Autodesk Inventor part; units mm, degrees
(part 2 of 2)
  line L911 (56.925, 86.925) -> (56.925, 75.1)
  line L912 (56.925, 75.1) -> (60.1, 75.1)
  line L913 (60.1, 75.1) -> (60.1, 64.9)
  line L914 (60.1, 64.9) -> (56.925, 64.9)
  line L915 (56.925, 64.9) -> (56.925, 55.1)
  line L916 (56.925, 55.1) -> (60.1, 55.1)
  line L917 (60.1, 55.1) -> (60.1, 44.9)
  line L918 (60.1, 44.9) -> (56.925, 44.9)
  line L919 (56.925, 44.9) -> (56.925, 35.1)
  line L920 (56.925, 35.1) -> (60.1, 35.1)
  line L921 (60.1, 35.1) -> (60.1, 24.9)
  line L922 (60.1, 24.9) -> (56.925, 24.9)
  line L923 (56.925, 24.9) -> (56.925, 15.1)
  line L924 (56.925, 15.1) -> (60.1, 15.1)
  line L925 (60.1, 15.1) -> (60.1, 4.9)
  line L926 (60.1, 4.9) -> (56.925, 4.9)
  line L927 (56.925, 4.9) -> (56.925, -4.9)
  line L928 (56.925, -4.9) -> (60.1, -4.9)
  line L929 (60.1, -4.9) -> (60.1, -15.1)
  line L930 (60.1, -15.1) -> (56.925, -15.1)
  line L931 (56.925, -15.1) -> (56.925, -24.9)
  line L932 (56.925, -24.9) -> (60.1, -24.9)
  line L933 (60.1, -24.9) -> (60.1, -35.1)
  line L934 (60.1, -35.1) -> (56.925, -35.1)
  line L935 (56.925, -35.1) -> (56.925, -44.9)
  line L936 (56.925, -44.9) -> (60.1, -44.9)
  line L937 (60.1, -44.9) -> (60.1, -55.1)
  line L938 (60.1, -55.1) -> (56.925, -55.1)
  line L939 (56.925, -55.1) -> (56.925, -64.9)
  line L940 (56.925, -64.9) -> (60.1, -64.9)
  line L941 (60.1, -64.9) -> (60.1, -75.1)
  line L942 (60.1, -75.1) -> (56.925, -75.1)
  line L943 (56.925, -75.1) -> (56.925, -86.925)
  line L944 (56.925, -86.925) -> (55.1, -86.925)
  line L945 (55.1, -86.925) -> (55.1, -90.1)
  line L946 (55.1, -90.1) -> (44.9, -90.1)
  line L947 (44.9, -90.1) -> (44.9, -86.925)
  line L948 (44.9, -86.925) -> (35.1, -86.925)
  line L949 (35.1, -86.925) -> (35.1, -90.1)
  line L950 (35.1, -90.1) -> (24.9, -90.1)
  line L951 (24.9, -90.1) -> (24.9, -86.925)
  line L952 (24.9, -86.925) -> (15.1, -86.925)
  line L953 (15.1, -86.925) -> (15.1, -90.1)
  line L954 (15.1, -90.1) -> (4.9, -90.1)
  line L955 (4.9, -90.1) -> (4.9, -86.925)
  line L956 (4.9, -86.925) -> (-4.9, -86.925)
  line L957 (-4.9, -86.925) -> (-4.9, -90.1)
  line L958 (-4.9, -90.1) -> (-15.1, -90.1)
  line L959 (-15.1, -90.1) -> (-15.1, -86.925)
  line L960 (-15.1, -86.925) -> (-24.9, -86.925)
  line L961 (-24.9, -86.925) -> (-24.9, -90.1)
  line L962 (-24.9, -90.1) -> (-35.1, -90.1)
  line L963 (-35.1, -90.1) -> (-35.1, -86.925)
  line L964 (-35.1, -86.925) -> (-44.9, -86.925)
  line L965 (-44.9, -86.925) -> (-44.9, -90.1)
  line L966 (-44.9, -90.1) -> (-55.1, -90.1)
  line L967 (-55.1, -90.1) -> (-55.1, -86.925)
  line L968 (-55.1, -86.925) -> (-56.925, -86.925)
  line L969 (-56.925, -86.925) -> (-56.925, -75.1)
  line L970 (-56.925, -75.1) -> (-60.1, -75.1)
  line L971 (-60.1, -75.1) -> (-60.1, -64.9)
  line L972 (-60.1, -64.9) -> (-56.925, -64.9)
  line L973 (-56.925, -64.9) -> (-56.925, -55.1)
  line L974 (-56.925, -55.1) -> (-60.1, -55.1)
  line L975 (-60.1, -55.1) -> (-60.1, -44.9)
  line L976 (-60.1, -44.9) -> (-56.925, -44.9)
  line L977 (-56.925, -44.9) -> (-56.925, -35.1)
  line L978 (-56.925, -35.1) -> (-60.1, -35.1)
  line L979 (-60.1, -35.1) -> (-60.1, -24.9)
  line L980 (-60.1, -24.9) -> (-56.925, -24.9)
  line L981 (-56.925, -24.9) -> (-56.925, -15.1)
  line L982 (-56.925, -15.1) -> (-60.1, -15.1)
  line L983 (-60.1, -15.1) -> (-60.1, -4.9)
  line L984 (-60.1, -4.9) -> (-56.925, -4.9)
  line L985 (-56.925, -4.9) -> (-56.925, 4.9)
  line L986 (-56.925, 4.9) -> (-60.1, 4.9)
  line L987 (-60.1, 4.9) -> (-60.1, 15.1)
  line L988 (-60.1, 15.1) -> (-56.925, 15.1)
  line L989 (-56.925, 15.1) -> (-56.925, 24.9)
  line L990 (-56.925, 24.9) -> (-60.1, 24.9)
  line L991 (-60.1, 24.9) -> (-60.1, 35.1)
  line L992 (-60.1, 35.1) -> (-56.925, 35.1)
  line L993 (-56.925, 35.1) -> (-56.925, 44.9)
  line L994 (-56.925, 44.9) -> (-60.1, 44.9)
  line L995 (-60.1, 44.9) -> (-60.1, 55.1)
  line L996 (-60.1, 55.1) -> (-56.925, 55.1)
  line L997 (-56.925, 55.1) -> (-56.925, 64.9)
  line L998 (-56.925, 64.9) -> (-60.1, 64.9)
  line L999 (-60.1, 64.9) -> (-60.1, 75.1)
  line L1000 (-60.1, 75.1) -> (-56.925, 75.1)
  line L1001 (-56.925, 75.1) -> (-56.925, 86.925)
  line L1002 (-56.925, 86.925) -> (-55.1, 86.925)
  line L1003 (-55.1, 86.925) -> (-55.1, 90.1)
  line L1004 (-55.1, 90.1) -> (-44.9, 90.1)
  line L1005 (-44.9, 90.1) -> (-44.9, 86.925)
  line L1006 (-44.9, 86.925) -> (-35.1, 86.925)
  line L1007 (-35.1, 86.925) -> (-35.1, 90.1)
  line L1008 (-35.1, 90.1) -> (-24.9, 90.1)
  line L1009 (-24.9, 90.1) -> (-24.9, 86.925)
  line L1010 (-24.9, 86.925) -> (-15.1, 86.925)
  line L1011 (-15.1, 86.925) -> (-15.1, 90.1)
  line L1012 (-14.9, 90.1) -> (-25.1, 90.1)
  line L1013 (-25.1, 90.1) -> (-25.1, 93.275)
  line L1014 (-25.1, 93.275) -> (-34.9, 93.275)
  line L1015 (-34.9, 93.275) -> (-34.9, 90.1)
  line L1016 (-34.9, 90.1) -> (-45.1, 90.1)
  line L1017 (-45.1, 90.1) -> (-45.1, 93.275)
  line L1018 (-45.1, 93.275) -> (-54.9, 93.275)
  line L1019 (-54.9, 93.275) -> (-54.9, 90.1)
  line L1020 (-54.9, 90.1) -> (-60.1, 90.1)
  line L1021 (-60.1, 90.1) -> (-60.1, 95.3)
  line L1022 (-60.1, 95.3) -> (-56.925, 95.3)
  line L1023 (-56.925, 95.3) -> (-56.925, 105.1)
  line L1024 (-56.925, 105.1) -> (-60.1, 105.1)
  line L1025 (-60.1, 105.1) -> (-60.1, 115.3)
  line L1026 (-60.1, 115.3) -> (-56.925, 115.3)
  line L1027 (-56.925, 115.3) -> (-56.925, 125.1)
  line L1028 (-56.925, 125.1) -> (-60.1, 125.1)
  line L1029 (-60.1, 125.1) -> (-60.1, 135.3)
  line L1030 (-60.1, 135.3) -> (-56.925, 135.3)
  line L1031 (-56.925, 135.3) -> (-56.925, 145.1)
  line L1032 (-56.925, 145.1) -> (-60.1, 145.1)
  line L1033 (-60.1, 145.1) -> (-60.1, 155.3)
  line L1034 (-60.1, 155.3) -> (-56.925, 155.3)
  line L1035 (-56.925, 155.3) -> (-56.925, 165.1)
  line L1036 (-56.925, 165.1) -> (-60.1, 165.1)
  line L1037 (-60.1, 165.1) -> (-60.1, 175.3)
  line L1038 (-60.1, 175.3) -> (-56.925, 175.3)
  line L1039 (-56.925, 175.3) -> (-56.925, 185.1)
  line L1040 (-56.925, 185.1) -> (-60.1, 185.1)
  line L1041 (-60.1, 185.1) -> (-60.1, 195.3)
  line L1042 (-60.1, 195.3) -> (-56.925, 195.3)
  line L1043 (-56.925, 195.3) -> (-56.925, 205.1)
  line L1044 (-56.925, 205.1) -> (-60.1, 205.1)
  line L1045 (-60.1, 205.1) -> (-60.1, 210.3)
  line L1046 (-60.1, 210.3) -> (-54.9, 210.3)
  line L1047 (-54.9, 210.3) -> (-54.9, 207.125)
  line L1048 (-54.9, 207.125) -> (-45.1, 207.125)
  line L1049 (-45.1, 207.125) -> (-45.1, 210.3)
  line L1050 (-45.1, 210.3) -> (-34.9, 210.3)
  line L1051 (-34.9, 210.3) -> (-34.9, 207.125)
  line L1052 (-34.9, 207.125) -> (-25.1, 207.125)
  line L1053 (-25.1, 207.125) -> (-25.1, 210.3)
  line L1054 (-25.1, 210.3) -> (-14.9, 210.3)
  line L1055 (-14.9, 210.3) -> (-14.9, 207.125)
  line L1056 (-14.9, 207.125) -> (-5.1, 207.125)
  line L1057 (-5.1, 207.125) -> (-5.1, 210.3)
  line L1058 (-5.1, 210.3) -> (5.1, 210.3)
  line L1059 (5.1, 210.3) -> (5.1, 207.125)
  line L1060 (5.1, 207.125) -> (14.9, 207.125)
  line L1061 (14.9, 207.125) -> (14.9, 210.3)
  line L1062 (14.9, 210.3) -> (25.1, 210.3)
  line L1063 (25.1, 210.3) -> (25.1, 207.125)
  line L1064 (25.1, 207.125) -> (34.9, 207.125)
  line L1065 (34.9, 207.125) -> (34.9, 210.3)
  line L1066 (34.9, 210.3) -> (45.1, 210.3)
  line L1067 (45.1, 210.3) -> (45.1, 207.125)
  line L1068 (45.1, 207.125) -> (54.9, 207.125)
  line L1069 (54.9, 207.125) -> (54.9, 210.3)
  line L1070 (54.9, 210.3) -> (60.1, 210.3)
  line L1071 (60.1, 210.3) -> (60.1, 205.1)
  line L1072 (60.1, 205.1) -> (56.925, 205.1)
  line L1073 (56.925, 205.1) -> (56.925, 195.3)
  line L1074 (56.925, 195.3) -> (60.1, 195.3)
  line L1075 (60.1, 195.3) -> (60.1, 185.1)
  line L1076 (60.1, 185.1) -> (56.925, 185.1)
  line L1077 (56.925, 185.1) -> (56.925, 175.3)
  line L1078 (56.925, 175.3) -> (60.1, 175.3)
  line L1079 (60.1, 175.3) -> (60.1, 165.1)
  line L1080 (60.1, 165.1) -> (56.925, 165.1)
  line L1081 (56.925, 165.1) -> (56.925, 155.3)
  line L1082 (56.925, 155.3) -> (60.1, 155.3)
  line L1083 (60.1, 155.3) -> (60.1, 145.1)
  line L1084 (60.1, 145.1) -> (56.925, 145.1)
  line L1085 (56.925, 145.1) -> (56.925, 135.3)
  line L1086 (56.925, 135.3) -> (60.1, 135.3)
  line L1087 (60.1, 135.3) -> (60.1, 125.1)
  line L1088 (60.1, 125.1) -> (56.925, 125.1)
  line L1089 (56.925, 125.1) -> (56.925, 115.3)
  line L1090 (56.925, 115.3) -> (60.1, 115.3)
  line L1091 (60.1, 115.3) -> (60.1, 105.1)
  line L1092 (60.1, 105.1) -> (56.925, 105.1)
  line L1093 (56.925, 105.1) -> (56.925, 95.3)
  line L1094 (56.925, 95.3) -> (60.1, 95.3)
  line L1095 (60.1, 95.3) -> (60.1, 90.1)
  line L1096 (60.1, 90.1) -> (54.9, 90.1)
  line L1097 (54.9, 90.1) -> (54.9, 93.275)
  line L1098 (54.9, 93.275) -> (45.1, 93.275)
  line L1099 (45.1, 93.275) -> (45.1, 90.1)
  line L1100 (45.1, 90.1) -> (34.9, 90.1)
  line L1101 (34.9, 90.1) -> (34.9, 93.275)
  line L1102 (34.9, 93.275) -> (25.1, 93.275)
  line L1103 (25.1, 93.275) -> (25.1, 90.1)
  line L1104 (25.1, 90.1) -> (14.9, 90.1)
  line L1105 (14.9, 90.1) -> (14.9, 93.275)
  line L1106 (14.9, 93.275) -> (5.1, 93.275)
  line L1107 (5.1, 93.275) -> (5.1, 90.1)
  line L1108 (5.1, 90.1) -> (-5.1, 90.1)
  line L1109 (-5.1, 90.1) -> (-5.1, 93.275)
  line L1110 (-5.1, 93.275) -> (-14.9, 93.275)
  line L1111 (-14.9, 93.275) -> (-14.9, 90.1)
  line L1112 (75.3, 90.1) -> (75.3, 86.925)
  line L1113 (75.3, 86.925) -> (85.1, 86.925)
  line L1114 (85.1, 86.925) -> (85.1, 90.1)
  line L1115 (85.1, 90.1) -> (95.3, 90.1)
  line L1116 (95.3, 90.1) -> (95.3, 86.925)
  line L1117 (95.3, 86.925) -> (105.1, 86.925)
  line L1118 (105.1, 86.925) -> (105.1, 90.1)
  line L1119 (105.1, 90.1) -> (115.3, 90.1)
  line L1120 (115.3, 90.1) -> (115.3, 86.925)
  line L1121 (115.3, 86.925) -> (125.1, 86.925)
  line L1122 (125.1, 86.925) -> (125.1, 90.1)
  line L1123 (125.1, 90.1) -> (135.3, 90.1)
  line L1124 (135.3, 90.1) -> (135.3, 86.925)
  line L1125 (135.3, 86.925) -> (145.1, 86.925)
  line L1126 (145.1, 86.925) -> (145.1, 90.1)
  line L1127 (145.1, 90.1) -> (155.3, 90.1)
  line L1128 (155.3, 90.1) -> (155.3, 86.925)
  line L1129 (155.3, 86.925) -> (165.1, 86.925)
  line L1130 (165.1, 86.925) -> (165.1, 90.1)
  line L1131 (165.1, 90.1) -> (175.3, 90.1)
  line L1132 (175.3, 90.1) -> (175.3, 86.925)
  line L1133 (175.3, 86.925) -> (180.3, 86.925)
  line L1134 (180.3, 86.925) -> (180.3, 74.9)
  line L1135 (180.3, 74.9) -> (177.125, 74.9)
  line L1136 (177.125, 74.9) -> (177.125, 65.1)
  line L1137 (177.125, 65.1) -> (180.3, 65.1)
  line L1138 (180.3, 65.1) -> (180.3, 54.9)
  line L1139 (180.3, 54.9) -> (177.125, 54.9)
  line L1140 (177.125, 54.9) -> (177.125, 45.1)
  line L1141 (177.125, 45.1) -> (180.3, 45.1)
  line L1142 (180.3, 45.1) -> (180.3, 34.9)
  line L1143 (180.3, 34.9) -> (177.125, 34.9)
  line L1144 (177.125, 34.9) -> (177.125, 25.1)
  line L1145 (177.125, 25.1) -> (180.3, 25.1)
  line L1146 (180.3, 25.1) -> (180.3, 14.9)
  line L1147 (180.3, 14.9) -> (177.125, 14.9)
  line L1148 (177.125, 14.9) -> (177.125, 5.1)
  line L1149 (177.125, 5.1) -> (180.3, 5.1)
  line L1150 (180.3, 5.1) -> (180.3, -5.1)
  line L1151 (180.3, -5.1) -> (177.125, -5.1)
  line L1152 (177.125, -5.1) -> (177.125, -14.9)
  line L1153 (177.125, -14.9) -> (180.3, -14.9)
  line L1154 (180.3, -14.9) -> (180.3, -25.1)
  line L1155 (180.3, -25.1) -> (177.125, -25.1)
  line L1156 (177.125, -25.1) -> (177.125, -34.9)
  line L1157 (177.125, -34.9) -> (180.3, -34.9)
  line L1158 (180.3, -34.9) -> (180.3, -45.1)
  line L1159 (180.3, -45.1) -> (177.125, -45.1)
  line L1160 (177.125, -45.1) -> (177.125, -54.9)
  line L1161 (177.125, -54.9) -> (180.3, -54.9)
  line L1162 (180.3, -54.9) -> (180.3, -65.1)
  line L1163 (180.3, -65.1) -> (177.125, -65.1)
  line L1164 (177.125, -65.1) -> (177.125, -74.9)
  line L1165 (177.125, -74.9) -> (180.3, -74.9)
  line L1166 (180.3, -74.9) -> (180.3, -86.925)
  line L1167 (180.3, -86.925) -> (175.3, -86.925)
  line L1168 (175.3, -86.925) -> (175.3, -90.1)
  line L1169 (175.3, -90.1) -> (165.1, -90.1)
  line L1170 (165.1, -90.1) -> (165.1, -86.925)
  line L1171 (165.1, -86.925) -> (155.3, -86.925)
  line L1172 (155.3, -86.925) -> (155.3, -90.1)
  line L1173 (155.3, -90.1) -> (145.1, -90.1)
  line L1174 (145.1, -90.1) -> (145.1, -86.925)
  line L1175 (145.1, -86.925) -> (135.3, -86.925)
  line L1176 (135.3, -86.925) -> (135.3, -90.1)
  line L1177 (135.3, -90.1) -> (125.1, -90.1)
  line L1178 (125.1, -90.1) -> (125.1, -86.925)
  line L1179 (125.1, -86.925) -> (115.3, -86.925)
  line L1180 (115.3, -86.925) -> (115.3, -90.1)
  line L1181 (115.3, -90.1) -> (105.1, -90.1)
  line L1182 (105.1, -90.1) -> (105.1, -86.925)
  line L1183 (105.1, -86.925) -> (95.3, -86.925)
  line L1184 (95.3, -86.925) -> (95.3, -90.1)
  line L1185 (95.3, -90.1) -> (85.1, -90.1)
  line L1186 (85.1, -90.1) -> (85.1, -86.925)
  line L1187 (85.1, -86.925) -> (75.3, -86.925)
  line L1188 (75.3, -86.925) -> (75.3, -90.1)
  line L1189 (75.3, -90.1) -> (65.1, -90.1)
  line L1190 (65.1, -90.1) -> (65.1, -86.925)
  line L1191 (65.1, -86.925) -> (60.1, -86.925)
  line L1192 (60.1, -86.925) -> (60.1, -74.9)
  line L1193 (60.1, -74.9) -> (63.275, -74.9)
  line L1194 (63.275, -74.9) -> (63.275, -65.1)
  line L1195 (63.275, -65.1) -> (60.1, -65.1)
  line L1196 (60.1, -65.1) -> (60.1, -54.9)
  line L1197 (60.1, -54.9) -> (63.275, -54.9)
  line L1198 (63.275, -54.9) -> (63.275, -51.4)
  line L1199 (63.275, -51.4) -> (65.475, -51.4)
  line L1200 (65.475, -51.4) -> (65.475, -52.65)
  line L1201 (65.475, -52.65) -> (67.775, -52.65)
  line L1202 (67.775, -52.65) -> (67.775, -51.4)
  line L1203 (67.775, -51.4) -> (74.1, -51.4)
  line L1204 (74.1, -51.4) -> (74.1, -48.6)
  line L1205 (74.1, -48.6) -> (67.775, -48.6)
  line L1206 (67.775, -48.6) -> (67.775, -47.35)
  line L1207 (67.775, -47.35) -> (65.475, -47.35)
  line L1208 (65.475, -47.35) -> (65.475, -48.6)
  line L1209 (65.475, -48.6) -> (63.275, -48.6)
  line L1210 (63.275, -48.6) -> (63.275, -45.1)
  line L1211 (63.275, -45.1) -> (60.1, -45.1)
  line L1212 (60.1, -45.1) -> (60.1, -34.9)
  line L1213 (60.1, -34.9) -> (63.275, -34.9)
  line L1214 (63.275, -34.9) -> (63.275, -25.1)
  line L1215 (63.275, -25.1) -> (60.1, -25.1)
  line L1216 (60.1, -25.1) -> (60.1, -14.9)
  line L1217 (60.1, -14.9) -> (63.275, -14.9)
  line L1218 (63.275, -14.9) -> (63.275, -5.1)
  line L1219 (63.275, -5.1) -> (60.1, -5.1)
  line L1220 (60.1, -5.1) -> (60.1, 5.1)
  line L1221 (60.1, 5.1) -> (63.275, 5.1)
  line L1222 (63.275, 5.1) -> (63.275, 14.9)
  line L1223 (63.275, 14.9) -> (60.1, 14.9)
  line L1224 (60.1, 14.9) -> (60.1, 25.1)
  line L1225 (60.1, 25.1) -> (63.275, 25.1)
  line L1226 (63.275, 25.1) -> (63.275, 34.9)
  line L1227 (63.275, 34.9) -> (60.1, 34.9)
  line L1228 (60.1, 34.9) -> (60.1, 45.1)
  line L1229 (60.1, 45.1) -> (63.275, 45.1)
  line L1230 (63.275, 45.1) -> (63.275, 48.6)
  line L1231 (63.275, 48.6) -> (65.475, 48.6)
  line L1232 (65.475, 48.6) -> (65.475, 47.35)
  line L1233 (65.475, 47.35) -> (67.775, 47.35)
  line L1234 (67.775, 47.35) -> (67.775, 48.6)
  line L1235 (67.775, 48.6) -> (74.1, 48.6)
  line L1236 (74.1, 48.6) -> (74.1, 51.4)
  line L1237 (74.1, 51.4) -> (67.775, 51.4)
  line L1238 (67.775, 51.4) -> (67.775, 52.65)
  line L1239 (67.775, 52.65) -> (65.475, 52.65)
  line L1240 (65.475, 52.65) -> (65.475, 51.4)
  line L1241 (65.475, 51.4) -> (63.275, 51.4)
  line L1242 (63.275, 51.4) -> (63.275, 54.9)
  line L1243 (63.275, 54.9) -> (60.1, 54.9)
  line L1244 (60.1, 54.9) -> (60.1, 65.1)
  line L1245 (60.1, 65.1) -> (63.275, 65.1)
  line L1246 (63.275, 65.1) -> (63.275, 74.9)
  line L1247 (63.275, 74.9) -> (60.1, 74.9)
  line L1248 (60.1, 74.9) -> (60.1, 86.925)
  line L1249 (60.1, 86.925) -> (65.1, 86.925)
  line L1250 (65.1, 86.925) -> (65.1, 90.1)
  line L1251 (65.1, 90.1) -> (75.3, 90.1)
  line L1252 (43.7, -59.9) -> (43.7, 59.9)
  line L1253 (43.7, 59.9) -> (-43.7, 59.9)
  line L1254 (-43.7, 59.9) -> (-43.7, -59.9)
  line L1255 (-43.7, -59.9) -> (43.7, -59.9)
  circle A22 centre (-67.924, -59.1479) radius 1.078 projected
  circle A23 centre (-102.924, -59.1479) radius 1.078 projected
  point P0 (0, 0)
  dimension "d8" = 0.1
  dimension "d9" = 0.1
  dimension "d10" = 0.1
  dimension "d11" = 0.1
  dimension "d12" = 0.1
  dimension "d13" = 0.1
  dimension "d14" = 0.1
  dimension "d15" = 0.1
  constraints: 1248 end point, 616 other
  measures "d8" distance between parallel lines of L8 L632
  measures "d9" distance between parallel lines of L0 L748
  measures "d10" distance between parallel lines of L6 L752
  measures "d11" distance between parallel lines of L188 L756
  measures "d12" distance between parallel lines of L377 L896
  measures "d13" distance between parallel lines of L448 L1012
  measures "d14" distance between parallel lines of L589 L1112
  measures "d15" distance between parallel lines of L268 L1252
extrude "Extrusion2" add sketch "Sketch2" along normal blind 3.175 contours L632 L633 L634 L635 L636 L637 L638 L639 L640 L641 L642 L643 L644 L645 L646 L647 L648 L649 L650 L651 L652 L653 L654 L655 L656 L657 L658 L659 L660 L661 L662 L663 L664 L665 L666 L667 L668 L669 L670 L671 L672 L673 L674 L675 L676 L677 L678 L679 L680 L681 L682 L683 L684 L685 L686 L687 L688 L689 L690 L691 L692 L693 L694 L695 L696 L697 L698 L699 L700 L701 L702 L703 L704 L705 L706 L707 L708 L709 L710 L711 L712 L713 L714 L715 L716 L717 L718 L719 L720 L721 L722 L723 L724 L725 L726 L727 L728 L729 L730 L731 L732 L733 L734 L735 L736 L737 L738 L739 L740 L741 L742 L743 L744 L745 L746 L747 | L891 L892 L893 L894 L895 L756 L757 L758 L759 L760 L761 L762 L763 L764 L765 L766 L767 L768 L769 L770 L771 L772 L773 L774 L775 L776 L777 L778 L779 L780 L781 L782 L783 L784 L785 L786 L787 L788 L789 L790 L791 L792 L793 L794 L795 L796 L797 L798 L799 L800 L801 L802 L803 L804 L805 L806 L807 L808 L809 L810 L811 L812 L813 L814 L815 L816 L817 L818 L819 L820 L821 L822 L823 L824 L825 L826 L827 L828 L829 L830 L831 L832 L833 L834 L835 L836 L837 L838 L839 L840 L841 L842 L843 L844 L845 L846 L847 L848 L849 L850 L851 L852 L853 L854 L855 L856 L857 L858 L859 L688 L860 L861 L862 L863 L684 L864 L865 L866 L867 L680 L868 L869 L870 L871 L676 L872 L873 L874 L875 L672 L876 L877 L878 L879 L668 L880 L881 L882 L883 L664 L884 L885 L886 L887 L660 L888 L889 L890 | L1000 L1001 L1002 L1003 L1004 L1005 L1006 L1007 L1008 L1009 L1010 L1011 L896 L897 L898 L899 L900 L901 L902 L903 L904 L905 L906 L907 L908 L909 L910 L911 L912 L913 L914 L915 L916 L917 L918 L919 L920 L921 L922 L923 L924 L925 L926 L927 L928 L929 L930 L931 L932 L933 L934 L935 L936 L937 L938 L939 L940 L941 L942 L943 L944 L945 L946 L947 L948 L949 L950 L951 L952 L953 L954 L955 L956 L957 L958 L959 L960 L961 L962 L963 L964 L965 L966 L967 L968 L969 L970 L833 L971 L829 L972 L973 L974 L975 L813 L976 L977 L978 L979 L809 L980 L981 L982 L983 L805 L984 L985 L986 L987 L801 L988 L989 L990 L991 L797 L992 L993 L994 L995 L781 L996 L997 L998 L999 L777 | L1020 L1021 L1022 L1023 L1024 L1025 L1026 L1027 L1028 L1029 L1030 L1031 L1032 L1033 L1034 L1035 L1036 L1037 L1038 L1039 L1040 L1041 L1042 L1043 L1044 L1045 L1046 L1047 L1048 L1049 L1050 L1051 L1052 L1053 L1054 L1055 L1056 L1057 L1058 L1059 L1060 L1061 L1062 L1063 L1064 L1065 L1066 L1067 L1068 L1069 L1070 L1071 L1072 L1073 L1074 L1075 L1076 L1077 L1078 L1079 L1080 L1081 L1082 L1083 L1084 L1085 L1086 L1087 L1088 L1089 L1090 L1091 L1092 L1093 L1094 L1095 L1096 L908 L1097 L1098 L1099 L1100 L904 L1101 L1102 L1103 L1104 L900 L1105 L1106 L1107 L1108 L896 L1109 L1110 L1111 L1012 L1008 L1013 L1014 L1015 L1016 L1004 L1017 L1018 L1019 | L1248 L1249 L1250 L1251 L1112 L1113 L1114 L1115 L1116 L1117 L1118 L1119 L1120 L1121 L1122 L1123 L1124 L1125 L1126 L1127 L1128 L1129 L1130 L1131 L1132 L1133 L1134 L1135 L1136 L1137 L1138 L1139 L1140 L1141 L1142 L1143 L1144 L1145 L1146 L1147 L1148 L1149 L1150 L1151 L1152 L1153 L1154 L1155 L1156 L1157 L1158 L1159 L1160 L1161 L1162 L1163 L1164 L1165 L1166 L1167 L1168 L1169 L1170 L1171 L1172 L1173 L1174 L1175 L1176 L1177 L1178 L1179 L1180 L1181 L1182 L1183 L1184 L1185 L1186 L1187 L1188 L1189 L1190 L1191 L1192 L941 L1193 L1194 L1195 L1196 L937 L1197 L1198 L1199 L1200 L1201 L1202 L1203 L1204 L1205 L1206 L1207 L1208 L1209 L1210 L1211 L1212 L933 L1213 L1214 L1215 L1216 L929 L1217 L1218 L1219 L1220 L925 L1221 L1222 L1223 L1224 L921 L1225 L1226 L1227 L1228 L917 L1229 L1230 L1231 L1232 L1233 L1234 L1235 L1236 L1237 L1238 L1239 L1240 L1241 L1242 L1243 L1244 L913 L1245 L1246 L1247 | A22 | A23
equation "\"d8\" = laserKerf"
equation "\"d9\" = laserKerf"
equation "\"d10\" = laserKerf"
equation "\"d11\" = laserKerf"
equation "\"d12\" = laserKerf"
equation "\"d13\" = laserKerf"
equation "\"d14\" = laserKerf"
equation "\"d15\" = laserKerf"
equation "\"d16\" = materialThickness"
equation "\"materialThickness\" = 3.175"
equation "\"laserKerf\" = 0.1"
equation "\"cardPinDiameter\" = 3"
equation "\"centeralShaftDiameter\" = 8"
equation "\"cardWidth\" = 85.6"
equation "\"cardHeight\" = 53.98"
equation "\"cardThickness\" = 0.76"
equation "\"cardFillet\" = 2.88"
equation "\"cardClearence\" = 0.5"
equation "\"bearingOd\" = 22"
equation "\"bearingWidth\" = 8"
equation "\"axleHeight\" = 95"
equation "\"nutTrapClearence\" = 2"
equation "\"nutTrapwidth\" = 5.5"
equation "\"nutTrapDepth\" = 2.5"
equation "\"magnetDiameter\" = 6"
equation "\"magnetLength\" = 3"
equation "\"magnetProtusion\" = 0.25"
equation "\"spoolThickness\" = 5.588"
body "Solid2"
